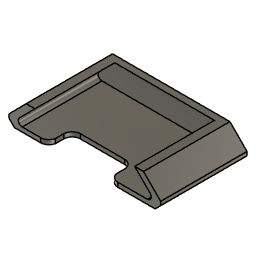
Slidey AUX v1_0 (Autodesk Fusion 360 design; units mm, degrees)
Autodesk Fusion 360 part; units mm, degrees
note: some values were not read from the file. Chosen so that the rebuilt part matches the saved one: which pieces of a blend or face edit are solid.
sketch "Sketch4" plane through (0, 0, 0) normal (0, 0, 1) x (1, 0, 0)
  line L0 (-20, 5) -> (-14, 5)
  line L1 (-14, 5) -> (-14, 45)
  line L2 (-14, 45) -> (-20, 45)
  line L3 (-20, 45) -> (-20, 5)
  line L4 (-25, 0) -> (-9, 0)
  line L5 (-9, 0) -> (-9, 50)
  line L6 (-9, 50) -> (-25, 50)
  line L7 (-25, 50) -> (-25, 0)
  line L8 (-25, 0) -> (-27, 17.5)
  line L9 (-45, 17.5) -> (-47, 0)
  line L10 (-45, 17.5) -> (-27, 17.5)
  line L11 (-27, 17.5) -> (-27, 33)
  line L12 (-27, 33) -> (-45, 33)
  line L13 (-45, 33) -> (-45, 17.5)
  line L14 (-27, 33) -> (-25, 50)
  line L15 (-63, 50) -> (-63, 0)
  line L16 (-47, 50) -> (-63, 50)
  line L17 (-47, 0) -> (-47, 50)
  line L18 (-52, 45) -> (-58, 45)
  line L19 (-52, 5) -> (-52, 45)
  line L20 (-58, 45) -> (-58, 5)
  line L21 (-63, 0) -> (-47, 0)
  line L22 (-58, 5) -> (-52, 5)
  line L23 (-45, 33) -> (-47, 50)
  dimension "d32" = 18
  constraint horizontal L0
  constraint perpendicular L0 L1
  constraint perpendicular L1 L2
  constraint perpendicular L0 L3
  constraint perpendicular L1 L4
  constraint perpendicular L4 L5
  constraint perpendicular L5 L6
  constraint perpendicular L4 L7
  constraint horizontal L22
  constraint perpendicular L19 L22
  constraint perpendicular L18 L19
  constraint perpendicular L20 L22
  constraint perpendicular L19 L21
  constraint perpendicular L17 L21
  constraint perpendicular L16 L17
  constraint perpendicular L15 L21
  measures "d32" distance of L8.end L9.start
extrude "Extrude3" add sketch "Sketch4" along normal blind 2 contours L9 L13 L17 L23 | L15 L16 L17 L21 makes body 1
extrude "Extrude5" add sketch "Sketch4" along normal blind 2 separate body contours L4 L5 L6 L7 | L7 L8 L11 L14 makes body 2
extrude "Extrude6" add sketch "Sketch4" along normal blind 2 contours L10 L11 L12 L13 bodies 1 2
fillet "Fillet4" radius 5 8 edges at (-63, 0, 1) (-47, 0, 1) (-63, 50, 1) (-47, 50, 1) (-25, 50, 1) (-9, 50, 1) (-9, 0, 1) (-25, 0, 1) on bodies 1 2
fillet "Fillet4" radius 2.5 8 edges at (-52, 5, 1) (-58, 45, 1) (-52, 45, 1) (-58, 5, 1) (-20, 45, 1) (-14, 45, 1) (-14, 5, 1) (-20, 5, 1) on bodies 1 2
sketch "Sketch5" plane through (0, 17.5, 0) normal (0, -1, 0) x (1, 0, 0)
  line L0 (-45, 2) -> (-48.9997, 6)
  line L1 (-48.9997, 6) -> (-22.9997, 6)
  line L2 (-22.9997, 6) -> (-27, 2)
  line L3 (-27, 2) -> (-45, 2)
  line L4 (-45, 0) -> (-27, 0)
  line L5 (-27, 2) -> (-45, 2)
  line L6 (-27, 0) -> (-27, 2)
  line L7 (-45, 2) -> (-45, 0)
  dimension "d98" = 18
  constraint horizontal L1
  constraint perpendicular L0 L2
  constraint parallel L1 L3
  constraint coincident L0.start L3.end
  measures "d98" distance of L2.end L0.start
extrude "Extrude4" add sketch "Sketch5" against normal blind 14.4 contours L0 L1 L2 L3 L5 bodies 1
sketch "Sketch15" plane through (0, 0, 6) normal (0, 0, 1) x (-1, 0, 0)
  line L0 (48.9997, -17.5) -> (22.9997, -17.5)
  line L1 (22.9997, -17.5) -> (22.9997, -31.9)
  line L2 (22.9997, -31.9) -> (48.9997, -31.9)
  line L3 (48.9997, -31.9) -> (48.9997, -17.5)
  line L4 (48.9997, -31.9) -> (22.9997, -31.9)
  line L5 (22.9997, -17.5) -> (48.9997, -17.5)
  line L6 (48.9997, -31.9) -> (48.9997, -17.5)
  line L7 (22.9997, -31.9) -> (22.9997, -17.5)
  line L8 (48.9997, -31.9) -> (44.9997, -31.9)
  line L9 (44.9997, -31.9) -> (26.9997, -31.9)
  line L10 (44.9929, -17.5) -> (26.9929, -17.5)
  line L11 (44.9997, -31.9) -> (44.9997, -18.7)
  line L12 (44.9997, -18.7) -> (26.9997, -18.7)
  line L13 (26.9997, -18.7) -> (26.9997, -31.9)
  line L14 (39.1742, -31.9) -> (29.5, -31.9)
  line L15 (29.4997, -18.7) -> (29.5, -17.5)
  line L16 (41.9997, -31.9) -> (41.9997, -18.7)
  line L17 (26.9997, -31.9) -> (26.9997, -29.9)
  line L18 (26.9997, -29.9) -> (41.9997, -29.9)
  line L19 (26.9997, -29.9) -> (26.9997, -26.4)
  line L20 (26.9997, -26.4) -> (31.9997, -26.4)
  line L21 (31.9997, -26.4) -> (31.9997, -29.9)
  line L22 (26.9997, -18.7) -> (26.9997, -20.7)
  line L23 (26.9997, -20.7) -> (28.9997, -20.7)
  line L24 (28.9997, -20.7) -> (28.9997, -18.7)
  line L25 (29.4997, -18.7) -> (29.4997, -21.7)
  line L26 (29.4997, -21.7) -> (40.4997, -21.7)
  line L27 (40.4997, -21.7) -> (40.4997, -18.7)
  line L28 (40.4997, -18.7) -> (40.5, -17.5)
  dimension "d66" = 26
  dimension "d67" = 14.4
  dimension "d68" = 4
  dimension "d69" = 18
  dimension "d70" = 18
  dimension "d72" = 13.2
  dimension "d73" = 18
  dimension "d124" = 3
  dimension "d125" = 3
  dimension "d126" = 2
  dimension "d127" = 3.5
  dimension "d128" = 5
  dimension "d129" = 2
  dimension "d130" = 2
  dimension "d135" = 3
  dimension "d136" = 11
  dimension "d137" = 1.2
  constraint coincident L2.end L3.start
  constraint coincident L1.end L2.start
  constraint coincident L0.end L1.start
  constraint coincident L0.start L3.end
  constraint perpendicular L6 L8
  constraint parallel L4 L9
  constraint coincident L5 L10.start
  constraint coincident L5 L10.end
  constraint perpendicular L10 L11
  constraint perpendicular L11 L12
  constraint coincident L4 L14.start
  constraint coincident L4 L14.end
  constraint coincident L12 L15.start
  constraint coincident L5 L15.end
  constraint coincident L10 L15.end
  constraint coincident L9 L16.start
  constraint coincident L12 L16.end
  constraint perpendicular L12 L16
  constraint coincident L13 L17.end
  constraint coincident L16 L18.end
  constraint perpendicular L16 L18
  constraint perpendicular L18 L19
  constraint perpendicular L13 L20
  constraint perpendicular L20 L21
  constraint perpendicular L12 L22
  constraint perpendicular L22 L23
  constraint coincident L12 L24.end
  constraint perpendicular L12 L24
  constraint perpendicular L12 L25
  constraint perpendicular L25 L26
  constraint coincident L12 L27.end
  constraint perpendicular L12 L27
  constraint coincident L10 L28.end
  measures "d66" distance of L2.end L1.end
  measures "d67" distance of L2.end L0.start
  measures "d68" distance of L2.end L8.end
  measures "d69" distance of L8.end L9.end
  measures "d70" distance of L10.start L10.end
  measures "d72" distance of L8.end L11.end
  measures "d73" distance of L11.end L12.end
  measures "d124" distance of L8.end L16.start
  measures "d125" distance of L11 L16
  measures "d126" distance of L9.end L17.end
  measures "d127" distance of L17.end L19.end
  measures "d128" distance of L19.end L20.end
  measures "d129" distance of L12.end L22.end
  measures "d130" distance of L22.end L23.end
  measures "d135" distance of L15.start L25.end
  measures "d136" distance of L25.end L26.end
  measures "d137" vertical distance of L15.start L15.end
extrude "Extrude23" cut sketch "Sketch15" against normal blind 1.7 contours L2 L4 L9 L11 L12 L16 | L2 L4 L9 L13 L14 L16 L17 L18 | L12 L13 L22 L23 L24 | L13 L18 L19 L20 L21 bodies 1
extrude "Extrude24" cut sketch "Sketch15" against normal blind 2.9 contours L12 L25 L26 L27 | L12 L13 L16 L18 L20 L21 L23 L24 L25 L26 L27 bodies 1
sketch "Sketch16" plane through (0, 31.9, 0) normal (0, 1, 0) x (-1, 0, 0)
  line L0 (26.9997, 6) -> (22.9997, 6)
  line L1 (22.9997, 6) -> (27, 2)
  line L2 (45, 2) -> (48.9997, 6)
  line L3 (48.9997, 6) -> (44.9997, 6)
  line L4 (45, 2) -> (46.6, 2)
  line L5 (46.6, 2) -> (50.2, 5.6166)
  line L6 (27, 2) -> (25.4, 2)
  line L7 (25.4, 2) -> (21.8, 5.6515)
  line L8 (27, 2) -> (22.9997, 6)
  line L9 (45, 2) -> (48.9997, 6)
  line L10 (44.9997, 6) -> (44.9995, 6.1042)
  line L11 (26.9997, 6) -> (26.9996, 6.0732)
  line L12 (44.9997, 6) -> (48.9997, 6)
  line L13 (26.9997, 4.3) -> (26.9997, 6)
  line L14 (44.9997, 6) -> (44.9997, 4.3)
  line L15 (44.9997, 4.3) -> (26.9997, 4.3)
  line L16 (22.9997, 6) -> (48.9997, 6)
  line L17 (48.9997, 6) -> (48.9997, 6.8)
  line L18 (50.2, 5.6166) -> (50.2, 6.8)
  line L19 (21.8, 5.6515) -> (21.8, 6.8)
  line L20 (21.8, 6.8) -> (50.2, 6.8)
  line L21 (27, 2) -> (45, 2)
  dimension "d85" = 1.6
  dimension "d86" = 1.6
  constraint coincident L2.start L4.start
  constraint coincident L1.end L6.start
  constraint coincident L0.end L1.start
  constraint coincident L2.end L3.start
  constraint coincident L3.end L10.start
  constraint coincident L0.start L11.start
  constraint perpendicular L12 L17
  constraint vertical L18
  constraint perpendicular L16 L19
  constraint perpendicular L18 L20
  measures "d85" distance of L2.start L4.end
  measures "d86" distance of L1.end L6.end
extrude "Extrude18" add sketch "Sketch16" against normal blind 14.4 separate body contours L0 L1 L3 L6 L7 L8 L12 L16 L17 L19 L20 | L2 L4 L5 L9 L17 L18 L20 makes body 3
sketch "Sketch17" plane through (0, 0, 6.8) normal (0, 0, 1) x (-1, 0, 0)
  line L0 (-31.9, -21.7724) -> (-31.9, -50.1726)
  line L1 (-31.9, -50.1726) -> (-17.5, -50.1726)
  line L2 (-17.5, -50.1726) -> (-17.5, -21.7724)
  line L3 (-17.5, -21.7724) -> (-31.9, -21.7724)
  line L4 (-31.9, -21.7724) -> (-33.1, -21.7724)
  line L5 (-31.9, -50.1726) -> (-33.1, -50.1726)
  line L6 (-33.1, -50.1726) -> (-33.1, -21.7724)
  line L7 (-31.9, -21.7724) -> (-31.9, -50.1726)
  line L8 (21.8, -31.9) -> (50.2, -31.9)
  line L9 (50.2, -31.9) -> (50.2, -17.5)
  line L10 (50.2, -17.5) -> (21.8, -17.5)
  line L11 (21.8, -17.5) -> (21.8, -31.9)
  dimension "d92" = 1.2
  constraint coincident L0.start L3.end
  constraint perpendicular L0 L4
  constraint coincident L0.end L1.start
  constraint perpendicular L0 L5
  measures "d92" distance of L0.end L5.end
sketch "Sketch18" plane through (0, 17.5, 0) normal (0, -1, 0) x (1, 0, 0)
  line L0 (-25.4, 2) -> (-21.8, 5.6515)
  line L1 (-50.2, 5.6166) -> (-46.6, 2)
  line L2 (-46.6, 2) -> (-45, 2)
  line L3 (-44.9997, 7) -> (-44.9997, 6)
  line L4 (-26.9997, 6) -> (-26.9997, 7)
  line L5 (-26.9997, 7) -> (-44.9997, 7)
  line L6 (-44.9997, 6) -> (-26.9997, 6)
  line L7 (-21.8, 5.6515) -> (-21.8, 6.8)
  line L8 (-21.8, 6.8) -> (-50.2, 6.8)
  line L9 (-50.2, 6.8) -> (-50.2, 5.6166)
  line L10 (-22.9997, 6) -> (-27, 2)
  line L11 (-27, 2) -> (-25.4, 2)
  line L12 (-45, 2) -> (-48.9997, 6)
  line L13 (-48.9997, 6) -> (-22.9997, 6)
extrude "Extrude21" add sketch "Sketch16" along normal blind 1.2 bodies 3
extrude "Extrude25" cut sketch "Sketch15" along normal blind 1 contours L0 L5 L10 L12 L15 L28 | L12 L25 L26 L27 bodies 3
fillet "Fillet7" radius 1.5 2 edges at (-40.4997, 21.7, 6.4) (-29.4997, 21.7, 6.4) on bodies 3
fillet "Fillet7" radius 1.5 2 edges at (-40.5, 17.5, 6.4) (-29.5, 17.5, 6.4) on bodies 3
fillet "Fillet8" radius 0.8 2 edges at (-48.9997, 24.7, 6) (-22.9997, 24.7, 6) on bodies 1
fillet "Fillet9" radius 0.7 2 edges at (-22.9997, 24.7, 6) (-48.9997, 24.7, 6) on bodies 3
move_face "OffsetFaces8" offset -0.5 4 faces at (-50.2, 22.7, 6.4055) (-21.8, 27.9, 6.0344) (-50.2, 22.7, 6.4055) (-21.8, 27.9, 6.0344) on bodies 3
chamfer "Chamfer14" distance 1 angle 45 4 edges at (-22.3, 25.3, 6.8) (-49.7, 25.3, 6.8) (-22.3, 25.3, 6.8) (-49.7, 25.3, 6.8) on bodies 3
move_body "Move2" bodies 3 to x (-1, 0, 0) y (0, 1, 0) z (0, 0, -1) at (-21.9, 0, 6.8)
hidden bodies 1
